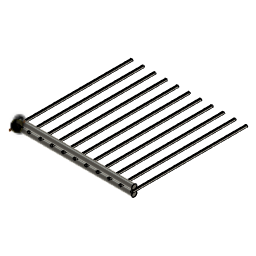
LED Strip Mount (Autodesk Fusion 360 archive; units mm, degrees)
design "Elfa shelf"
Autodesk Fusion 360 part; units mm, degrees
note: some values were not read from the file. Chosen so that the rebuilt part matches the saved one: which bodies a step acts on.
sketch "Small Wire" plane through (0, 0, 0) normal (0, 1, 0) x (1, 0, 0)
  line L0 (-0.5, -1.05) -> (0.5, -1.05)
  line L1 (0.5, -1.05) -> (-0.5, -1.05)
  line L2 (-0.5, -1.05) -> (0.5, -1.05)
  line L3 (-0.5, 1.05) -> (0.5, 1.05)
  arc A0 (0.5, -1.05) -> (0.5, 1.05) centre (0.5, 0) ccw
  arc A1 (-0.5, 1.05) -> (-0.5, -1.05) centre (-0.5, 0) ccw
  arc A2 (14.5, -1.05) -> (14.5, 1.05) centre (14.5, 0) ccw
  line L4 (14.5, -1.05) -> (13.5, -1.05)
  line L5 (13.5, 1.05) -> (14.5, 1.05)
  arc A3 (13.5, 1.05) -> (13.5, -1.05) centre (13.5, 0) ccw
  line L6 (13.5, -1.05) -> (14.5, -1.05)
  line L7 (13.5, -1.05) -> (14.5, -1.05)
  arc A4 (28.5, -1.05) -> (28.5, 1.05) centre (28.5, 0) ccw
  line L8 (28.5, -1.05) -> (27.5, -1.05)
  line L9 (27.5, 1.05) -> (28.5, 1.05)
  arc A5 (27.5, 1.05) -> (27.5, -1.05) centre (27.5, 0) ccw
  line L10 (27.5, -1.05) -> (28.5, -1.05)
  line L11 (27.5, -1.05) -> (28.5, -1.05)
  arc A6 (42.5, -1.05) -> (42.5, 1.05) centre (42.5, 0) ccw
  line L12 (42.5, -1.05) -> (41.5, -1.05)
  line L13 (41.5, 1.05) -> (42.5, 1.05)
  arc A7 (41.5, 1.05) -> (41.5, -1.05) centre (41.5, 0) ccw
  line L14 (41.5, -1.05) -> (42.5, -1.05)
  line L15 (41.5, -1.05) -> (42.5, -1.05)
  arc A8 (56.5, -1.05) -> (56.5, 1.05) centre (56.5, 0) ccw
  line L16 (56.5, -1.05) -> (55.5, -1.05)
  line L17 (55.5, 1.05) -> (56.5, 1.05)
  arc A9 (55.5, 1.05) -> (55.5, -1.05) centre (55.5, 0) ccw
  line L18 (55.5, -1.05) -> (56.5, -1.05)
  line L19 (55.5, -1.05) -> (56.5, -1.05)
  arc A10 (70.5, -1.05) -> (70.5, 1.05) centre (70.5, 0) ccw
  line L20 (70.5, -1.05) -> (69.5, -1.05)
  line L21 (69.5, 1.05) -> (70.5, 1.05)
  arc A11 (69.5, 1.05) -> (69.5, -1.05) centre (69.5, 0) ccw
  line L22 (69.5, -1.05) -> (70.5, -1.05)
  line L23 (69.5, -1.05) -> (70.5, -1.05)
  arc A12 (84.5, -1.05) -> (84.5, 1.05) centre (84.5, 0) ccw
  line L24 (84.5, -1.05) -> (83.5, -1.05)
  line L25 (83.5, 1.05) -> (84.5, 1.05)
  arc A13 (83.5, 1.05) -> (83.5, -1.05) centre (83.5, 0) ccw
  line L26 (83.5, -1.05) -> (84.5, -1.05)
  line L27 (83.5, -1.05) -> (84.5, -1.05)
  arc A14 (98.5, -1.05) -> (98.5, 1.05) centre (98.5, 0) ccw
  line L28 (98.5, -1.05) -> (97.5, -1.05)
  line L29 (97.5, 1.05) -> (98.5, 1.05)
  arc A15 (97.5, 1.05) -> (97.5, -1.05) centre (97.5, 0) ccw
  line L30 (97.5, -1.05) -> (98.5, -1.05)
  line L31 (97.5, -1.05) -> (98.5, -1.05)
  arc A16 (112.5, -1.05) -> (112.5, 1.05) centre (112.5, 0) ccw
  line L32 (112.5, -1.05) -> (111.5, -1.05)
  line L33 (111.5, 1.05) -> (112.5, 1.05)
  arc A17 (111.5, 1.05) -> (111.5, -1.05) centre (111.5, 0) ccw
  line L34 (111.5, -1.05) -> (112.5, -1.05)
  line L35 (111.5, -1.05) -> (112.5, -1.05)
  arc A18 (126.5, -1.05) -> (126.5, 1.05) centre (126.5, 0) ccw
  line L36 (126.5, -1.05) -> (125.5, -1.05)
  line L37 (125.5, 1.05) -> (126.5, 1.05)
  arc A19 (125.5, 1.05) -> (125.5, -1.05) centre (125.5, 0) ccw
  line L38 (125.5, -1.05) -> (126.5, -1.05)
  line L39 (125.5, -1.05) -> (126.5, -1.05)
  arc A20 (140.5, -1.05) -> (140.5, 1.05) centre (140.5, 0) ccw
  line L40 (140.5, -1.05) -> (139.5, -1.05)
  line L41 (139.5, 1.05) -> (140.5, 1.05)
  arc A21 (139.5, 1.05) -> (139.5, -1.05) centre (139.5, 0) ccw
  line L42 (139.5, -1.05) -> (140.5, -1.05)
  line L43 (139.5, -1.05) -> (140.5, -1.05)
  point P0 (14, 0)
  point P1 (28, 0)
  point P2 (42, 0)
  point P3 (56, 0)
  point P4 (70, 0)
  point P5 (84, 0)
  point P6 (98, 0)
  point P7 (112, 0)
  point P8 (126, 0)
  point P9 (140, 0)
  dimension "d19" = 1
  dimension "d21" = 0.5
  dimension "d22" = 1
  dimension "d25" = 2.1
  dimension "d28" = 14
  dimension "d29" = 0
  constraint horizontal L0
  constraint horizontal L2
  constraint horizontal L3
  constraint equal L2 L3
  constraint tangent L2 A0
  constraint tangent L3 A0
  constraint tangent L2 A1
  measures "d19" distance of L0.start L0.end
  measures "d21" horizontal distance of origin L0.end
  measures "d22" distance of L0.end L0.start
  measures "d25" distance of L0.start L3.start
extrude "Extrude1" add sketch "Small Wire" along normal blind 140 makes body 1 at (139.1409, 93.3333, 0.9867) makes body 2 at (111.1409, 93.3333, 0.9867) makes body 3 at (83.1409, 93.3333, 0.9867) makes body 4 at (70.9437, 93.3333, 0.9516) makes body 5 at (27.4085, 93.3333, -1.046) makes body 6 at (124.6399, 93.3333, -0.6023) makes body 7 at (-1.1749, 93.3333, -0.8043) makes body 8 at (41.4085, 46.6667, -1.046) makes body 9 at (56.5915, 46.6667, 1.046) makes body 10 at (97.1409, 93.3333, 0.9867) makes body 11 at (13.1409, 93.3333, 0.9867)
sketch "Large Wire" plane through (0, 0, 0) normal (1, 0, 0) x (0, 1, 0)
  circle A0 centre (3.08, 3.745) radius 3.08
  circle A1 centre (3.08, -3.745) radius 3.08
  line L0 (0, -1.05) -> (0, 1.05) construction
  line L1 (8.9827, 0.665) -> (-8.9827, 0.665) construction
  line L2 (-8.9827, 0.665) -> (-8.9827, -0.665) construction
  line L3 (-8.9827, -0.665) -> (8.9827, -0.665) construction
  line L4 (8.9827, -0.665) -> (8.9827, 0.665) construction
  line L5 (8.9827, 0.665) -> (-8.9827, -0.665) construction
  line L6 (-8.9827, 0.665) -> (8.9827, -0.665) construction
  dimension "d11" = 6.16
  dimension "d12" = 6.16
  dimension "d14" = 1.33
  constraint tangent A0 L0
  constraint tangent A1 L0
  constraint horizontal L1
  constraint perpendicular L1 L2
  constraint parallel L1 L3
  constraint parallel L2 L4
  constraint coincident L5 origin
  constraint coincident L6 origin
  constraint tangent A1 L3
  constraint tangent A0 L1
  measures "d11" diameter of A0
  measures "d12" diameter of A1
  measures "d14" distance of L1.start L3.end
extrude "Extrude2" cut sketch "Large Wire" along normal blind 140 bodies 1 2 3 4 5 6 7 8 9 10
extrude "Extrude3" add sketch "Large Wire" 2 faces at (0, 3.4305, -0.82) (0, 2.7174, 0.9878) along normal blind 140 separate body on bodies 7 makes body 12 at (46.6667, 6.1447, -4.0517) makes body 13 at (93.3333, 6.1447, 4.0517)
equation "Spacing = 14 mm"
equation "Small_Wire = 2.1 mm"
equation "Large_Wire = 6.16 mm"
equation "d9 = Spacing * 10"
equation "d11 = Large_Wire"
equation "d12 = Large_Wire"
equation "Rail_Height = 13.65 mm"
equation "d14 = Rail_Height - 2 * Large_Wire"
equation "d15 = Spacing * 10"
equation "d17 = Spacing * 10"
equation "d25 = Small_Wire"
equation "d28 = Spacing"
